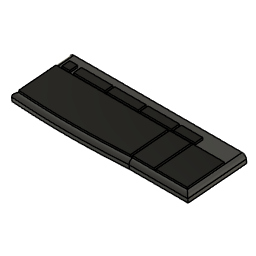
Keyboard-V1 (Autodesk Fusion 360 design; units mm, degrees)
Autodesk Fusion 360 part; units mm, degrees
note: some values were not read from the file. Chosen so that the rebuilt part matches the saved one: which bodies a step acts on.
sketch "Skizze1" plane through (0, 0, 0) normal (0, 0, 1) x (1, 0, 0)
  line L0 (-87.2456, 47.6268) -> (362.7544, 47.6268)
  line L1 (362.7544, 47.6268) -> (362.7544, -102.3732)
  line L2 (362.7544, -102.3732) -> (-87.2456, -102.3732)
  line L3 (-87.2456, -102.3732) -> (-87.2456, 47.6268)
  spline S0 degree 5 poles (-87.2456, -102.3732) (-81.4378, -102.7546) (-69.8054, -103.4839) (-52.306, -104.477) (-28.8703, -105.5965) (0.6079, -106.6318) (30.2855, -107.2713) (60.1783, -107.484) (90.2934, -107.2558) (120.6205, -106.6068) (151.143, -105.5702) (175.7042, -104.4568) (194.2005, -103.4722) (206.5643, -102.7504) (212.7544, -102.3732) knots 0 0 0 0 0 0 0.1 0.2 0.3 0.4 0.5 0.6 0.7 0.8 0.9 1 1 1 1 1 1
  point P0 (212.7544, -102.3732)
  point P1 (57.7544, -102.3732)
  point P2 (57.7544, -102.3732)
  point P3 (57.7544, -107.3732)
  point P4 (57.7544, -102.3732)
  point P5 (57.7544, -107.3732)
  dimension "d1" = 450
  dimension "d2" = 150
  dimension "d3" = 150
  dimension "d4" = 305
  dimension "d6" = 5
  constraint horizontal L0
  constraint vertical L1
  constraint horizontal L2
  constraint vertical L3
  constraint coincident L2 P0
  constraint coincident L2 P4
  constraint coincident P4 P2
  constraint coincident P5 P3
  constraint coincident P0 S0.end
  measures "d1" distance of L0.start L0.end
  measures "d2" distance of L0.start L2.end
  measures "d3" distance of L1.end P0
  measures "d4" distance of L1.end P4
  measures "d6" distance of P4 P5
extrude "Extrusion1" add sketch "Skizze1" along normal blind 20 makes body 1
move_body "Verschieben1" bodies 1 to x (1, 0, 0) y (0, 0.984808, 0.173648) z (0, -0.173648, 0.984808) at (0, 4.1965, -7.9665)
move_body "Verschieben2" bodies 1 to x (1, 0, 0) y (0, 0.996195, -0.087156) z (0, 0.087156, 0.996195) at (0, 0.2332, 3.9592)
move_body "Verschieben3" bodies 1 to x (1, 0, 0) y (0, 1, 0) z (0, 0, 1) at (0, 0, 15)
ref_plane "Arbeitsebene1" through (0, 0, 0) normal (0, 0, 1) x (1, 0, 0)
move_body "Verschieben4" bodies 1 to x (1, 0, 0) y (0, 1, 0) z (0, 0, 1) at (0, 0, -1.735)
sketch "Skizze2" plane through (0, -0.7464, 8.5316) normal (0, 0.087156, -0.996195) x (-1, 0, 0)
  line L0 (87.2456, -97.8903) -> (87.2456, 52.1097)
  line L1 (87.2456, 52.1097) -> (-362.7544, 52.1097)
  line L2 (-362.7544, 52.1097) -> (-362.7544, -97.8903)
  line L3 (-362.7544, -97.8903) -> (-212.7544, -97.8903)
  spline S0 degree 5 poles (87.2456, -97.8903) (81.4378, -98.2717) (69.8054, -99.0009) (52.306, -99.9941) (28.8703, -101.1136) (-0.6079, -102.1489) (-30.2855, -102.7884) (-60.1783, -103.0011) (-90.2934, -102.7728) (-120.6205, -102.1239) (-151.143, -101.0873) (-175.7042, -99.9739) (-194.2005, -98.9893) (-206.5643, -98.2675) (-212.7544, -97.8903) knots 0 0 0 0 0 0 0.1 0.2 0.3 0.4 0.5 0.6 0.7 0.8 0.9 1 1 1 1 1 1
  line L4 (52.2456, 37.1097) -> (72.2456, 37.1097)
  line L5 (72.2456, 37.1097) -> (72.2456, 31.1097)
  line L6 (72.2456, 31.1097) -> (52.2456, 31.1097)
  line L7 (52.2456, 31.1097) -> (52.2456, 37.1097)
  line L8 (-347.7544, 37.1097) -> (-327.7544, 37.1097)
  line L9 (-327.7544, 37.1097) -> (-327.7544, 31.1097)
  line L10 (-327.7544, 31.1097) -> (-347.7544, 31.1097)
  line L11 (-347.7544, 31.1097) -> (-347.7544, 37.1097)
  dimension "d10" = 20
  dimension "d11" = 6
  dimension "d12" = 15
  dimension "d13" = 15
  dimension "d14" = 20
  dimension "d15" = 6
  dimension "d16" = 15
  dimension "d17" = 15
  constraint horizontal L4
  constraint vertical L5
  constraint horizontal L6
  constraint vertical L7
  constraint horizontal L8
  constraint vertical L9
  constraint horizontal L10
  constraint vertical L11
  measures "d10" distance of L4.start L4.end
  measures "d11" distance of L4.start L6.end
  measures "d12" distance of L0 L5
  measures "d13" distance of L1 L4
  measures "d14" distance of L8.start L8.end
  measures "d15" distance of L8.start L10.end
  measures "d16" distance of L2 L11
  measures "d17" distance of L1 L8
extrude "Extrusion2" add sketch "Skizze2" along normal blind 50 separate body contours L4 L5 L6 L7 | L8 L9 L10 L11 makes body 2 at (341.0878, 39.1273, -21.4405) makes body 3 at (-58.9122, 39.1273, -21.4405)
split "Teilen1" by plane through (0, 0, 0) normal (0, 0, 1) bodies 3 2 makes body 4 at (341.0878, 36.5652, 7.844) makes body 5 at (-58.9122, 36.5652, 7.844)
delete_body "Körper entfernen1" bodies 3
delete_body "Körper entfernen2" bodies 2
fillet "Abrundung1" radius 10 4 edges at (60.2337, -104.9891, 19.488) (287.7544, -100.0073, 19.9238) (362.7544, -25.2927, 26.4605) (-87.2456, -25.2927, 26.4605) on bodies 1
sketch "Skizze3" plane through (0, -2.4895, 28.4555) normal (0, -0.087156, 0.996195) x (1, 0, 0)
  line L0 (352.7544, -87.8903) -> (352.7544, 52.1097)
  line L1 (352.7544, 52.1097) -> (-77.2456, 52.1097)
  line L2 (-77.2456, 52.1097) -> (-77.2456, -88.5075)
  spline S0 degree 3 poles (212.45, -87.8903) (212.3487, -87.8965) (212.2474, -87.9026) (212.1462, -87.9088) (186.8564, -89.45) (161.5477, -90.6815) (110.9036, -92.4036) (85.5679, -92.8848) (60.2312, -92.8911) (35.7425, -92.8973) (11.2541, -92.4566) (-34.5749, -90.8686) (-55.9188, -89.8259) (-77.2456, -88.5075) knots -29.925696 -29.925696 -29.925696 -29.925696 -29.895254 -29.895254 -29.895254 -22.29425 -22.29425 -14.693247 -14.693247 -14.693247 -7.346624 -7.346624 -0.93637 -0.93637 -0.93637 -0.93637
  line L3 (212.45, -87.8903) -> (352.7544, -87.8903)
  line L4 (352.7544, 32.1097) -> (-77.2456, 32.1097)
  line L5 (-77.2456, 12.1097) -> (352.7544, 12.1097)
  line L6 (-67.2456, 32.1097) -> (-67.2456, 12.1097)
  line L7 (-47.2456, 32.1097) -> (-47.2456, 12.1097)
  line L8 (-37.2456, 32.1097) -> (-37.2456, 12.1097)
  line L9 (272.7544, 32.1097) -> (272.7544, 12.1097)
  line L10 (217.7544, 32.1097) -> (217.7544, 12.1097)
  line L11 (212.7544, 32.1097) -> (212.7544, 12.1097)
  line L12 (42.7544, 32.1097) -> (42.7544, 12.1097)
  line L13 (47.7544, 32.1097) -> (47.7544, 12.1097)
  line L14 (127.7544, 32.1097) -> (127.7544, 12.1097)
  line L15 (132.7544, 32.1097) -> (132.7544, 12.1097)
  line L16 (-77.2456, 7.1097) -> (352.7544, 7.1097)
  line L17 (352.7544, 7.1097) -> (272.7544, 7.1097)
  line L18 (272.7544, 7.1097) -> (272.7544, -87.8903)
  line L19 (272.7544, -87.8903) -> (352.7544, -87.8903)
  line L20 (352.7544, -87.8903) -> (352.7544, 7.1097)
  line L21 (267.7544, 7.1097) -> (267.7544, -87.8903)
  line L22 (212.7544, 7.1097) -> (212.7544, -87.8903)
  line L23 (207.7544, 7.1097) -> (207.7544, -88.1732)
  dimension "d22" = -20
  dimension "d23" = 20
  dimension "d24" = 10
  dimension "d25" = 20
  dimension "d26" = 10
  dimension "d27" = 80
  dimension "d28" = 55
  dimension "d29" = 5
  dimension "d31" = 80
  dimension "d32" = 80
  dimension "d33" = 5
  dimension "d37" = 5
  dimension "d38" = 80
  dimension "d39" = 5
  dimension "d40" = 80
  dimension "d41" = 95
  dimension "d42" = 5
  dimension "d44" = 55
  dimension "d45" = 5
  constraint coincident L2 L5.start
  constraint coincident L0 L5.end
  constraint perpendicular L0 L5
  constraint coincident L4 L6.start
  constraint coincident L5 L6.end
  constraint perpendicular L5 L6
  constraint coincident L4 L7.start
  constraint coincident L5 L7.end
  constraint perpendicular L5 L7
  constraint coincident L4 L8.start
  constraint coincident L5 L8.end
  constraint perpendicular L5 L8
  constraint coincident L4 L9.start
  constraint coincident L5 L9.end
  constraint perpendicular L5 L9
  constraint coincident L4 L10.start
  constraint coincident L5 L10.end
  constraint perpendicular L5 L10
  constraint coincident L4 L11.start
  constraint coincident L5 L11.end
  constraint perpendicular L5 L11
  constraint coincident L4 L12.start
  constraint coincident L5 L12.end
  constraint perpendicular L5 L12
  constraint coincident L4 L13.start
  constraint coincident L5 L13.end
  constraint perpendicular L5 L13
  constraint coincident L4 L14.start
  constraint coincident L5 L14.end
  constraint perpendicular L5 L14
  constraint coincident L4 L15.start
  constraint coincident L5 L15.end
  constraint perpendicular L5 L15
  constraint coincident L2 L16.start
  constraint coincident L0 L16.end
  constraint perpendicular L0 L16
  constraint horizontal L17
  constraint vertical L18
  constraint horizontal L19
  constraint vertical L20
  constraint coincident L16 L21.start
  constraint coincident L3 L21.end
  constraint perpendicular L3 L21
  constraint coincident L16 L22.start
  constraint coincident L3 L22.end
  constraint perpendicular L3 L22
  constraint coincident L16 L23.start
  constraint coincident S0 L23.end
  constraint perpendicular L16 L23
  measures "d23" distance of L4 L5
  measures "d24" distance of L2 L6
  measures "d25" distance of L6 L7
  measures "d26" distance of L7 L8
  measures "d27" distance of L0 L9
  measures "d28" distance of L9 L10
  measures "d29" distance of L10 L11
  measures "d31" distance of L8 L12
  measures "d32" distance of L13 L14
  measures "d33" distance of L12 L13
  measures "d37" distance of L14 L15
  measures "d38" distance of L11 L15
  measures "d39" distance of L5 L16
  measures "d40" distance of L16.end L17.end
  measures "d41" distance of L16.end L0.start
  measures "d42" distance of L18 L21
  measures "d44" distance of L21 L22
  measures "d45" distance of L22 L23
extrude "Extrusion3" add sketch "Skizze3" along normal blind 0.5 contours L0 L3 L16 L17 L18 L19 L20 bodies 1
extrude "Extrusion4" cut 1 faces at (299.4211, -26.9966, 26.8133) along direction (0, 0.087156, -0.996195) blind 0.5 on bodies 1 bodies 1
extrude "Extrusion5" add sketch "Skizze3" along normal blind 5 separate body contours L0 L3 L16 L17 L18 L19 L20 | L3 L16 L21 L22 | L4 L5 L9 L10 | L4 L5 L11 L15 | L2 S0 L16 L23 | L4 L5 L6 L7 | L4 L5 L13 L14 | L4 L5 L8 L12 makes body 6 at (-60.5789, 22.8567, 30.673) makes body 7 at (249.4211, -58.4992, 23.5553) makes body 8 at (64.2056, -28.6132, 26.17) makes body 9 at (186.0878, 16.2154, 30.092) makes body 10 at (-10.5789, 22.8567, 30.673) makes body 11 at (299.4211, -26.953, 26.3152) makes body 12 at (74.4211, 16.2154, 30.092) makes body 13 at (236.0878, 16.2154, 30.092)
named bodies: "body", "leg-2", "leg-1"
